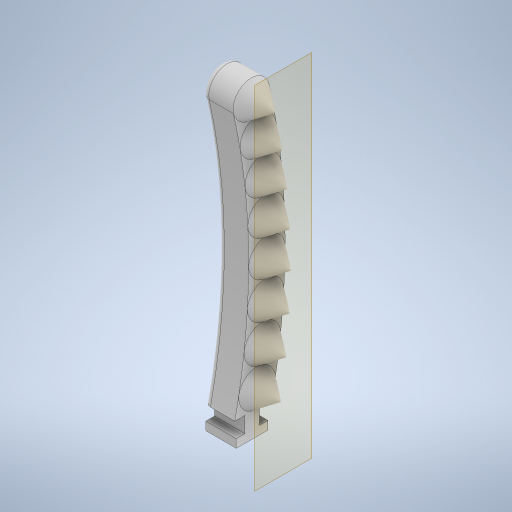
# Autodesk Inventor part: rake_arm
Saved by Autodesk Inventor 2023 (Build 270158000, 158)
## iProperties
Created: 2025-12-21
Part Number: rake_arm
Material: Generic
Document SubType Name: Modeling
Designer: Justin Pascual
Density: 1 g/cm^3
Appearance: Default
Author: Justin Pascual
Autodesk Inventor part; units mm, degrees
ref_plane "YZ Plane" through (0, 0, 0) normal (1, 0, 0) x (0, 1, 0)
ref_plane "XZ Plane" through (0, 0, 0) normal (0, 1, 0) x (-1, 0, 0)
ref_plane "XY Plane" through (0, 0, 0) normal (0, 0, 1) x (1, 0, 0)
sketch "Sketch1" plane through (0, 0, 0) normal (1, 0, 0) x (0, 1, 0)
  arc A0 (0, 0) -> (2.54, -0.5582) centre (57.15, 254) ccw construction
  arc A1 (117.6454, -14.8683) -> (114.3, 0) centre (115.9727, -7.4341) ccw
  line L0 (0, 0) -> (0, -15.5992) construction
  arc A2 (0, -15.5992) -> (2.54, -16.1251) centre (57.15, 254) ccw construction
  line L1 (0, -7.7996) -> (0, -10.8476) construction
  line L2 (2.54, -10.8476) -> (-4.064, -10.8476)
  line L3 (-4.064, -10.8476) -> (-4.064, -14.4036)
  line L4 (-4.064, -14.4036) -> (-7.62, -14.4036)
  line L5 (-7.62, -14.4036) -> (-7.62, -7.7996)
  line L6 (2.54, -7.7996) -> (-7.62, -7.7996) construction
  line L7 (0, -7.7996) -> (0, -4.7516) construction
  line L8 (2.54, -4.7516) -> (-4.064, -4.7516)
  line L9 (-4.064, -4.7516) -> (-4.064, -1.1956)
  line L10 (-4.064, -1.1956) -> (-7.62, -1.1956)
  line L11 (-7.62, -1.1956) -> (-7.62, -7.7996)
  line L12 (0, -7.7996) -> (2.54, -7.7996) construction
  line L13 (2.54, -0.5582) -> (2.54, -4.7516)
  line L14 (2.54, -10.8476) -> (2.54, -16.1251)
  arc A3 (2.54, -16.1251) -> (117.6454, -14.8683) centre (57.15, 254) ccw
  arc A4 (2.54, -0.5582) -> (114.3, 0) centre (57.15, 254) ccw
  point P0 (57.15, -6.35)
  point P1 (0, -10.8476)
  point P2 (0, -4.7516)
  dimension "d0" = 57.15
  dimension "d1" = 114.3
  dimension "d3" = 6.35
  dimension "d8" = 3.048
  dimension "d9" = 6.604
  dimension "d10" = 3.556
  dimension "d11" = 3.556
  dimension "d56" = 2.54
  constraints: 30 end point, 12 point on circle, 5 centre point, 4 symmetric about line, 3 perpendicular, 2 vertical, 1 coincident, 1 horizontal, 1 tangent
  measures "d0" horizontal distance of point (57.15, -6.35) A1.end
  measures "d1" distance of A1.end L0.start
  measures "d3" vertical distance of A1.end point (57.15, -6.35)
  measures "d8" distance of L1.start L1.end
  measures "d9" distance of L2.start L2.end
  measures "d10" distance of L2.end L3.end
  measures "d11" distance of L3.end L4.end
  measures "d56" distance of L12.start L12.end
extrude "Extrusion2" add sketch "Sketch1" along normal blind 12.7
sketch "Sketch2" plane through (12.7, 0, 0) normal (1, 0, 0) x (0, 0, -1)
  arc A0 (14.8683, 117.6454) -> (0, 114.3) centre (7.4341, 115.9727) ccw projected
  line L0 (7.4341, 115.9727) -> (14.8683, 117.6454) construction
  line L1 (7.4341, 115.9727) -> (9.1068, 108.5385) construction
  arc A1 (0, 0) -> (0, 114.3) centre (-254, 57.15) ccw projected
  arc A2 (15.5992, 0) -> (14.8683, 117.6454) centre (-254, 57.15) ccw projected
  arc A3 (6.3347, -6.3619) -> (7.4341, 115.9727) centre (-254, 57.15) ccw construction
  line L2 (9.1068, 108.5385) -> (11.4949, 93.4868) construction
  circle A4 centre (7.4341, 115.9727) radius 7.62
  circle A5 centre (10.3554, 101.0153) radius 7.62
  circle A6 centre (13.9648, 55.4874) radius 7.62
  circle A7 centre (12.0441, 25.0804) radius 7.62
  circle A8 centre (13.437, 40.2566) radius 7.62
  circle A9 centre (13.626, 70.7237) radius 7.62
  circle A10 centre (12.4215, 85.916) radius 7.62
  circle A11 centre (9.7907, 10.0079) radius 7.62
  dimension "d14" = 7.62
  dimension "d16" = 15.24
  dimension "d17" = 15.24
  dimension "d18" = 15.24
  dimension "d19" = 15.24
  dimension "d20" = 15.24
  dimension "d21" = 15.24
  dimension "d22" = 15.24
  constraints: 15 tangent, 9 centre point, 6 end point, 3 point on circle, 1 coincident, 1 concentric
  measures "d14" distance of L0.start L1.end
  measures "d16" diameter of A5
  measures "d17" diameter of A6
  measures "d18" diameter of A7
  measures "d19" diameter of A8
  measures "d20" diameter of A9
  measures "d21" diameter of A10
  measures "d22" diameter of A11
ref_plane "Work Plane1" through (22.86, 0, 0) normal (1, 0, 0) x (0, 0, -1)
sketch "Sketch3" plane through (22.86, 0, 0) normal (1, 0, 0) x (0, 0, -1)
  circle A0 centre (7.4341, 115.9727) radius 7.62 construction
  circle A1 centre (10.3554, 101.0153) radius 7.62 construction
  circle A2 centre (12.4215, 85.916) radius 7.62 construction
  circle A3 centre (13.626, 70.7237) radius 7.62 construction
  circle A4 centre (13.9648, 55.4874) radius 7.62 construction
  circle A5 centre (13.437, 40.2566) radius 7.62 construction
  circle A6 centre (12.0441, 25.0804) radius 7.62 construction
  circle A7 centre (9.7907, 10.0079) radius 7.62 construction
  point P0 (0, 0)
  constraints: 8 coincident
loft "Loft1" add profiles "Sketch2" section 2 point at (22.86, 115.9727, -7.4341) contours A4 A0
loft "Loft2" add profiles "Sketch2" section 2 point at (22.86, 101.0153, -10.3554) contours A5
loft "Loft3" add profiles "Sketch2" section 2 point at (22.86, 85.916, -12.4215) contours A10
loft "Loft4" add profiles "Sketch2" section 2 point at (22.86, 70.7237, -13.626) contours A9
loft "Loft5" add profiles "Sketch2" section 2 point at (22.86, 55.4874, -13.9648) contours A6
loft "Loft6" add profiles "Sketch2" section 2 point at (22.86, 40.2566, -13.437) contours A8
loft "Loft7" add profiles "Sketch2" section 2 point at (22.86, 25.0804, -12.0441) contours A7
loft "Loft8" add profiles "Sketch2" section 1 point at (22.86, 10.0079, -9.7907) contours A11
fillet "Fillet1" radius 2.54 3 edges at (0, 123.4068, -5.7615) (0, 60.159, -21.5736) (0, 58.4503, -6.3468)
equation "\"d0\" = 0.5 * d1"
body "Solid2"
